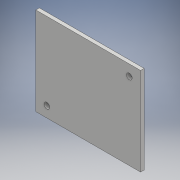
# Autodesk Inventor part: Lid
Saved by Autodesk Inventor 2017 (Build 210142000, 142)
## iProperties
Created: 2017-03-21
Part Number: Lid
Material: Generic
Document SubType Name: Modeling
Designer: Liam
Density: 1 g/cm^3
Appearance: Default
Author: Liam
Autodesk Inventor part; units mm, degrees
ref_plane "YZ Plane" through (0, 0, 0) normal (1, 0, 0) x (0, 1, 0)
ref_plane "XZ Plane" through (0, 0, 0) normal (0, 1, 0) x (-1, 0, 0)
ref_plane "XY Plane" through (0, 0, 0) normal (0, 0, 1) x (1, 0, 0)
sketch "Sketch1" plane through (0, 0, 0) normal (0, 1, 0) x (-1, 0, 0)
  line L0 (0, 0) -> (72.9, 0)
  line L1 (72.9, 0) -> (72.9, -61.3)
  line L2 (72.9, -61.3) -> (0, -61.3)
  line L3 (0, -61.3) -> (0, 0)
  dimension "d0" = 72.9
  dimension "d1" = 61.3
  constraints: 8 end point, 2 parallel, 1 horizontal, 1 perpendicular
  measures "d0" distance of L1.end L2.end
  measures "d1" distance of L0.end L1.end
extrude "Extrusion1" add sketch "Sketch1" along normal blind 2.5
sketch "Sketch2" plane through (0, 2.5, 0) normal (0, 1, 0) x (1, 0, 0)
  line L0 (-72.9, 0) -> (0, 0) projected
  line L1 (-72.9, 61.3) -> (-72.9, 0) projected
  line L2 (0, 61.3) -> (-72.9, 61.3) projected
  line L3 (0, 0) -> (0, 61.3) projected
  point P0 (-65.2, 53.8)
  point P1 (-7.8, 7.5)
  dimension "d6" = 7.7
  dimension "d7" = 7.5
  dimension "d8" = 7.5
  dimension "d9" = 7.8
  measures "d6" distance from line of point (-65.2, 53.8) L1
  measures "d7" distance from line of L2 point (-65.2, 53.8)
  measures "d8" distance from line of L0 point (-7.8, 7.5)
  measures "d9" distance from line of point (-7.8, 7.5) L3
hole "Hole1" at (-65.2, 2.5, -53.8) at (-7.8, 2.5, -7.5) direction (0, -1, 0) diameter 4 end through all
body "Solid1"
